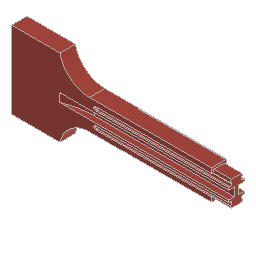
sentry (Autodesk Fusion 360 design; units mm, degrees)
Autodesk Fusion 360 part; units mm, degrees
sketch "base" plane through (0, 0, 0) normal (1, 0, 0) x (0, 1, 0)
  line L0 (0, 0) -> (0, 2.2125)
  line L1 (0, 0) -> (3.2, 0)
  line L2 (0, 2.2125) -> (1.175, 2.2125)
  line L3 (1.175, 2.2125) -> (1.175, 3.9625)
  line L4 (1.175, 3.9625) -> (0, 3.9625)
  line L5 (0, 3.9625) -> (0, 6.175)
  line L6 (0, 6.175) -> (3.2, 6.175)
  line L7 (3.2, 6.175) -> (3.2, 3.9625)
  line L8 (3.2, 3.9625) -> (2.025, 3.9625)
  line L9 (2.025, 3.9625) -> (2.025, 2.2125)
  line L10 (2.025, 2.2125) -> (3.2, 2.2125)
  line L11 (3.2, 2.2125) -> (3.2, 0)
  dimension "d1" = 2.2125
  dimension "d2" = 3.2
  dimension "d3" = 1.175
  dimension "d4" = 1.75
  dimension "d5" = 1.175
  dimension "d6" = 2.2125
  dimension "d7" = 3.2
  dimension "d8" = 2.2125
  dimension "d9" = 1.175
  dimension "d10" = 1.75
  dimension "d11" = 1.175
  constraint coincident L0.start L1.start
  constraint vertical L0
  constraint perpendicular L0 L1
  constraint perpendicular L0 L2
  constraint perpendicular L2 L3
  constraint perpendicular L3 L4
  constraint perpendicular L4 L5
  constraint perpendicular L5 L6
  constraint perpendicular L6 L7
  constraint perpendicular L7 L8
  constraint perpendicular L8 L9
  constraint perpendicular L9 L10
  measures "d1" distance of L0.start L0.end
  measures "d2" distance of L0.start L1.end
  measures "d3" distance of L0.end L2.end
  measures "d4" distance of L2.end L3.end
  measures "d5" distance of L3.end L4.end
  measures "d6" distance of L4.end L5.end
  measures "d7" distance of L5.end L6.end
  measures "d8" distance of L6.end L7.end
  measures "d9" distance of L7.end L8.end
  measures "d10" distance of L8.end L9.end
  measures "d11" distance of L9.end L10.end
extrude "Extrude1" add sketch "base" against normal blind 35
sketch "warding" plane through (0, 0, 0) normal (1, 0, 0) x (0, 1, 0)
  line L0 (0, 0) -> (3.2, 0) construction
  line L1 (0, 0) -> (0, 6.175) construction
  line L2 (0, 6.175) -> (3.2, 6.175) construction
  line L3 (0, 0) -> (0, 1) construction
  line L4 (3.2, 0) -> (3.2, 1) construction
  line L5 (0, 6.175) -> (0, 5.175) construction
  line L6 (3.2, 6.175) -> (3.2, 5.175) construction
  line L7 (0, 1) -> (0.6, 1)
  line L8 (3.2, 1) -> (2.6, 1)
  line L9 (0, 5.175) -> (0.6, 5.175)
  line L10 (3.2, 5.175) -> (2.6, 5.175)
  line L11 (0.6, 1) -> (0.6, 1.75)
  line L12 (2.6, 1) -> (2.6, 1.75)
  line L13 (0.6, 5.175) -> (0.6, 4.425)
  line L14 (2.6, 5.175) -> (2.6, 4.425)
  line L15 (0, 1) -> (0, 1.75)
  line L16 (3.2, 1) -> (3.2, 1.75)
  line L17 (0, 5.175) -> (0, 4.425)
  line L18 (3.2, 5.175) -> (3.2, 4.425)
  line L19 (0.6, 1.75) -> (0, 1.75)
  line L20 (3.2, 1.75) -> (2.6, 1.75)
  line L21 (0.6, 4.425) -> (0, 4.425)
  line L22 (2.6, 4.425) -> (3.2, 4.425)
  dimension "d14" = 3.2
  dimension "d15" = 6.175
  dimension "d16" = 3.2
  dimension "d17" = 1
  dimension "d18" = 1
  dimension "d19" = 1
  dimension "d20" = 1
  dimension "d21" = 0.6
  dimension "d22" = 0.6
  dimension "d23" = 0.6
  dimension "d24" = 0.6
  dimension "d25" = 0.75
  dimension "d26" = 0.75
  dimension "d27" = 0.75
  dimension "d28" = 0.75
  dimension "d29" = 0.75
  dimension "d30" = 0.75
  dimension "d31" = 0.75
  dimension "d32" = 0.75
  constraint coincident L0.start L1.start
  constraint horizontal L0
  constraint perpendicular L0 L1
  constraint perpendicular L1 L2
  constraint perpendicular L0 L3
  constraint perpendicular L0 L4
  constraint perpendicular L2 L5
  constraint perpendicular L2 L6
  constraint perpendicular L3 L7
  constraint perpendicular L4 L8
  constraint perpendicular L5 L9
  constraint perpendicular L6 L10
  constraint perpendicular L7 L11
  constraint perpendicular L8 L12
  constraint perpendicular L9 L13
  constraint perpendicular L10 L14
  constraint perpendicular L7 L15
  constraint perpendicular L8 L16
  constraint perpendicular L9 L17
  constraint perpendicular L10 L18
  measures "d14" distance of L0.start L0.end
  measures "d15" distance of L0.start L1.end
  measures "d16" distance of L1.end L2.end
  measures "d17" distance of L0.start L3.end
  measures "d18" distance of L0.end L4.end
  measures "d19" distance of L1.end L5.end
  measures "d20" distance of L2.end L6.end
  measures "d21" distance of L3.end L7.end
  measures "d22" distance of L4.end L8.end
  measures "d23" distance of L5.end L9.end
  measures "d24" distance of L6.end L10.end
  measures "d25" distance of L7.end L11.end
  measures "d26" distance of L8.end L12.end
  measures "d27" distance of L9.end L13.end
  measures "d28" distance of L10.end L14.end
  measures "d29" distance of L3.end L15.end
  measures "d30" distance of L4.end L16.end
  measures "d31" distance of L5.end L17.end
  measures "d32" distance of L6.end L18.end
extrude "Extrude2" cut sketch "warding" against normal blind 28
fillet "Fillet1" radius 0.325 8 edges at (-14, 0.6, 5.175) (-14, 0.6, 1.75) (-14, 0.6, 4.425) (-14, 0.6, 1) (-14, 2.6, 4.425) (-14, 2.6, 1) (-14, 2.6, 5.175) (-14, 2.6, 1.75)
fillet "Fillet2" radius 0.35 20 edges at (-28, 0.1375, 4.425) (-28, 0.5048, 4.5202) (-28, 0.6, 4.8) (-28, 0.5048, 5.0798) (-28, 0.1375, 5.175) (-28, 0.1375, 1) (-28, 0.5048, 1.0952) (-28, 0.6, 1.375) (-28, 0.5048, 1.6548) (-28, 0.1375, 1.75) (-28, 3.0625, 4.425) (-28, 2.6952, 4.5202) (-28, 2.6, 4.8) (-28, 2.6952, 5.0798) (-28, 3.0625, 5.175) (-28, 3.0625, 1) (-28, 2.6952, 1.0952) (-28, 2.6, 1.375) (-28, 2.6952, 1.6548) (-28, 3.0625, 1.75)
sketch "bow" plane through (-35, 0, 0) normal (-1, 0, 0) x (0, -1, 0)
  line L0 (-3.2, 0) -> (0, 0)
  line L1 (0, 0) -> (0, 2.2125)
  line L2 (0, 2.2125) -> (-1.175, 2.2125)
  line L3 (-1.175, 2.2125) -> (-1.175, 3.9625)
  line L4 (-1.175, 3.9625) -> (0, 3.9625)
  line L5 (0, 3.9625) -> (0, 6.175)
  line L6 (0, 6.175) -> (-3.2, 6.175)
  line L7 (-3.2, 6.175) -> (-3.2, 3.9625)
  line L8 (-3.2, 3.9625) -> (-2.025, 3.9625)
  line L9 (-2.025, 3.9625) -> (-2.025, 2.2125)
  line L10 (-2.025, 2.2125) -> (-3.2, 2.2125)
  line L11 (-3.2, 2.2125) -> (-3.2, 0)
  line L12 (0, 0) -> (0, 6.175) construction
  line L13 (0, 3.0875) -> (0, 11.0875)
  line L14 (0, 11.0875) -> (-3.2, 11.0875)
  line L15 (-3.2, 11.0875) -> (-3.2, -4.9125)
  line L16 (-3.2, -4.9125) -> (0, -4.9125)
  line L17 (0, -4.9125) -> (0, 6.175)
  dimension "d160" = 8
  dimension "d161" = 3.2
  dimension "d162" = 16
  dimension "d163" = 3.2
  constraint coincident L0.end L1.start
  constraint coincident L5.end L6.start
  constraint midpoint L12 L13.start
  constraint perpendicular L6 L13
  constraint perpendicular L13 L14
  constraint perpendicular L14 L15
  constraint perpendicular L15 L16
  measures "d160" distance of L13.start L13.end
  measures "d161" distance of L13.end L14.end
  measures "d162" distance of L14.end L15.end
  measures "d163" distance of L15.end L16.end
extrude "Extrude14" add sketch "bow" along normal blind 10
fillet "Fillet3" radius 6.25 2 edges at (-35, 1.6, 0) (-35, 1.6, 6.175)
fillet "Fillet4" radius 16.25 2 edges at (-35, 1.175, 3.0875) (-35, 2.025, 3.0875)
sketch "aws disc" plane through (0, 0, 0) normal (1, 0, 0) x (0, 1, 0)
  line L0 (0, 0) -> (1.6, 0) construction
  line L1 (1.6, 0) -> (1.6, 3.0875) construction
  line L2 (1.6, 3.0875) -> (1.6, 6.175) construction
  line L3 (1.6, 6.175) -> (0, 6.175) construction
  line L4 (1.6, 3.0875) -> (0, 3.0875) construction
  line L5 (1.6, 3.0875) -> (-0.2806, 3.9644) construction
  line L6 (1.6, 3.0875) -> (0, 3.0875) construction
  line L7 (-0.2806, 3.9644) -> (0.7502, 6.175)
  line L8 (1.6, 3.0875) -> (-0.2806, 2.2106) construction
  line L9 (1.6, 3.0875) -> (0, 3.0875) construction
  line L10 (-0.2806, 2.2106) -> (0.7502, 0)
  line L11 (1.6, 3.0875) -> (3.4806, 2.2106) construction
  line L12 (1.6, 3.0875) -> (3.4806, 3.9644) construction
  line L13 (3.4806, 3.9644) -> (2.4498, 6.175)
  line L14 (3.4806, 2.2106) -> (2.4498, 0)
  line L15 (0.7502, 6.175) -> (2.4498, 6.175)
  line L16 (0.7502, 0) -> (2.4498, 0)
  line L17 (-0.2806, 3.9644) -> (-0.2806, 2.2106)
  line L18 (3.4806, 3.9644) -> (3.4806, 2.2106)
  circle A0 centre (1.6, 3.0875) radius 4.25
  dimension "d37" = 1.6
  dimension "d38" = 3.0875
  dimension "d39" = 3.0875
  dimension "d40" = 1.6
  dimension "d41" = 1.6
  dimension "d42" = 25
  dimension "d43" = 2.075
  dimension "d44" = 25
  dimension "d45" = 2.075
  dimension "d46" = 8.5
  constraint coincident L0.start origin
  constraint horizontal L0
  constraint perpendicular L0 L1
  constraint parallel L1 L2
  constraint perpendicular L2 L3
  constraint perpendicular L1 L4
  constraint horizontal L6
  constraint coincident L3 L7.end
  constraint perpendicular L5 L7
  constraint horizontal L9
  constraint perpendicular L8 L10
  constraint equal L7 L10
  constraint parallel L5 L11
  constraint equal L5 L11
  constraint parallel L8 L12
  constraint equal L5 L12
  constraint perpendicular L12 L13
  constraint equal L7 L13
  constraint perpendicular L11 L14
  constraint equal L7 L14
  constraint coincident L1.end L2.start
  measures "d37" distance of L0.start L0.end
  measures "d38" distance of L0.end L1.end
  measures "d39" distance of L1.end L2.end
  measures "d40" distance of L2.end L3.end
  measures "d41" distance of L1.end L4.end
  measures "d42" angle of L5 L6
  measures "d43" distance of L1.end L5.end
  measures "d44" angle of L8 L9
  measures "d45" distance of L1.end L8.end
  measures "d46" diameter of A0
sketch "tip warding" plane through (0, 0, 0) normal (1, 0, 0) x (0, 1, 0)
  line L0 (0, 0) -> (3.2, 0)
  line L1 (1.6, 0) -> (1.6, 6.175) construction
  line L2 (1.6, 6.175) -> (0, 6.175)
  line L3 (1.6, 6.175) -> (3.2, 6.175)
  line L4 (0, 0) -> (0, 0.5)
  line L5 (3.2, 6.175) -> (3.2, 5.675)
  line L6 (0, 0.5) -> (3.2, 0.5)
  line L7 (3.2, 0.5) -> (3.2, 0)
  line L8 (3.2, 5.675) -> (0, 5.675)
  line L9 (0, 5.675) -> (0, 6.175)
  dimension "d47" = 3.2
  dimension "d48" = 6.175
  dimension "d49" = 1.6
  dimension "d50" = 1.6
  dimension "d51" = 0.5
  dimension "d52" = 0.5
  constraint coincident L0.start L4.start
  constraint horizontal L0
  constraint midpoint L0 L1.start
  constraint perpendicular L0 L1
  constraint perpendicular L1 L2
  constraint perpendicular L1 L3
  constraint perpendicular L0 L4
  constraint perpendicular L3 L5
  constraint perpendicular L4 L6
  constraint perpendicular L0 L7
  constraint perpendicular L5 L8
  constraint perpendicular L2 L9
  measures "d47" distance of L0.start L0.end
  measures "d48" distance of L1.start L1.end
  measures "d49" distance of L1.end L2.end
  measures "d50" distance of L1.end L3.end
  measures "d51" distance of L0.start L4.end
  measures "d52" distance of L3.end L5.end
extrude "Extrude3" cut sketch "tip warding" against normal blind 3.62
extrude "Extrude4" cut sketch "aws disc" against normal blind 3.62
sketch "Sketch12" plane through (0, 0, 0) normal (1, 0, 0) x (0, 1, 0)
  line L0 (0, 0) -> (1.6, 0) construction
  line L1 (1.6, 0) -> (1.6, 3.0875) construction
  line L2 (1.6, 3.0875) -> (0.6, 3.0875) construction
  line L3 (-0.6404, 3.4825) -> (3.8404, 2.6925) construction
  line L4 (-0.6404, 3.4825) -> (-0.0327, 6.9294)
  line L5 (3.8404, 2.6925) -> (3.2327, -0.7544)
  arc A0 (-0.6404, 3.4825) -> (-0.675, 3.0875) centre (1.6, 3.0875) ccw
  arc A1 (3.8404, 2.6925) -> (3.875, 3.0875) centre (1.6, 3.0875) ccw
  line L6 (3.875, 3.0875) -> (7.3391, 5.0875)
  line L7 (3.875, 3.0875) -> (1.6, 3.0875) construction
  line L8 (-0.675, 3.0875) -> (-4.1391, 1.0875)
  line L9 (-0.0327, 6.9294) -> (7.3391, 5.0875)
  line L10 (-4.1391, 1.0875) -> (3.2327, -0.7544)
  circle A2 centre (1.6, 3.0875) radius 7
  dimension "d197" = 1.6
  dimension "d198" = 3.0875
  dimension "d199" = 1
  dimension "d200" = 4.55
  dimension "d201" = 10
  dimension "d202" = 3.5
  dimension "d203" = 30
  dimension "d204" = 4
  dimension "d205" = 14
  constraint coincident L0.start origin
  constraint horizontal L0
  constraint perpendicular L0 L1
  constraint perpendicular L1 L2
  constraint midpoint L1.end L3
  constraint perpendicular L3 L4
  constraint perpendicular L3 L5
  constraint equal L4 L5
  constraint coincident L1.end L2.start
  constraint horizontal L1.end A0.end
  constraint collinear A0.end L1.end A1.end
  constraint horizontal L7
  constraint parallel L6 L8
  constraint equal L6 L8
  constraint concentric A1 A2
  measures "d197" distance of L0.start L0.end
  measures "d198" distance of L0.end L1.end
  measures "d199" distance of L1.end L2.end
  measures "d200" distance of L3.start L3.end
  measures "d201" angle of L2 L3
  measures "d202" distance of L3.start L4.end
  measures "d203" angle of L6 L7
  measures "d204" distance of A1.end L6.end
  measures "d205" diameter of A2
sketch "Sketch13" plane through (0, 0, 0) normal (1, 0, 0) x (0, 1, 0)
  circle A0 centre (1.6, 3.0875) radius 7
  line L0 (1.6, 3.0875) -> (0.6, 3.0875) construction
  line L1 (-0.6404, 3.4825) -> (3.8404, 2.6925) construction
  line L2 (-0.6404, 3.4825) -> (-0.0327, 6.9294)
  arc A1 (-0.6404, 3.4825) -> (-0.675, 3.0875) centre (1.6, 3.0875) ccw
  line L3 (-0.675, 3.0875) -> (-4.1391, 1.0875)
  line L4 (-0.675, 3.0875) -> (1.6, 3.0875) construction
  line L5 (3.8404, 2.6925) -> (3.2327, -0.7544)
  arc A2 (3.8404, 2.6925) -> (3.875, 3.0875) centre (1.6, 3.0875) ccw
  line L6 (3.875, 3.0875) -> (7.3391, 5.0875)
  line L7 (-0.0327, 6.9294) -> (7.3391, 5.0875)
  line L8 (-4.1391, 1.0875) -> (3.2327, -0.7544)
  dimension "d206" = 4.55
  dimension "d207" = 10
  dimension "d208" = 3.5
  dimension "d209" = 30
  dimension "d210" = 4
  constraint midpoint A0.centre L1
  constraint perpendicular L1 L2
  constraint coincident A0.centre L0.start
  constraint horizontal A0.centre A1.end
  constraint horizontal L4
  constraint perpendicular L1 L5
  constraint parallel L3 L6
  constraint equal L3 L6
  constraint collinear A0.centre A1.end A2.end
  constraint equal L2 L5
  measures "d206" distance of L1.start L1.end
  measures "d207" angle of L0 L1
  measures "d208" distance of L1.start L2.end
  measures "d209" angle of L3 L4
  measures "d210" distance of A1.end L3.end
sketch "Sketch14" plane through (0, 0, 0) normal (1, 0, 0) x (0, 1, 0)
  line L0 (1.6, 3.0875) -> (0.6, 3.0875) construction
  circle A0 centre (1.6, 3.0875) radius 7
  line L1 (-0.6404, 3.4825) -> (3.8404, 2.6925) construction
  line L2 (-0.6404, 3.4825) -> (-0.0327, 6.9294)
  arc A1 (-0.6404, 3.4825) -> (-0.675, 3.0875) centre (1.6, 3.0875) ccw
  line L3 (-0.675, 3.0875) -> (-4.1391, 1.0875)
  line L4 (-0.675, 3.0875) -> (1.6, 3.0875) construction
  line L5 (3.8404, 2.6925) -> (3.2327, -0.7544)
  arc A2 (3.8404, 2.6925) -> (3.875, 3.0875) centre (1.6, 3.0875) ccw
  line L6 (3.875, 3.0875) -> (7.3391, 5.0875)
  line L7 (-0.0327, 6.9294) -> (7.3391, 5.0875)
  line L8 (-4.1391, 1.0875) -> (3.2327, -0.7544)
  dimension "d211" = 4.55
  dimension "d212" = 10
  dimension "d213" = 3.5
  dimension "d214" = 30
  dimension "d215" = 4
  constraint midpoint L0.start L1
  constraint perpendicular L1 L2
  constraint coincident L0.start A0.centre
  constraint horizontal L0.start A1.end
  constraint horizontal L4
  constraint perpendicular L1 L5
  constraint equal L2 L5
  constraint collinear L0.start A1.end A2.end
  constraint parallel L3 L6
  constraint equal L3 L6
  measures "d211" distance of L1.start L1.end
  measures "d212" angle of L0 L1
  measures "d213" distance of L1.start L2.end
  measures "d214" angle of L3 L4
  measures "d215" distance of A1.end L3.end
sketch "Sketch15" plane through (0, 0, 0) normal (1, 0, 0) x (0, 1, 0)
  line L0 (1.6, 3.0875) -> (0.6, 3.0875) construction
  circle A0 centre (1.6, 3.0875) radius 7
  line L1 (-0.6404, 3.4825) -> (3.8404, 2.6925) construction
  line L2 (-0.6404, 3.4825) -> (-0.0327, 6.9294)
  arc A1 (-0.6404, 3.4825) -> (-0.675, 3.0875) centre (1.6, 3.0875) ccw
  line L3 (-0.675, 3.0875) -> (-4.1391, 1.0875)
  line L4 (-0.675, 3.0875) -> (1.6, 3.0875) construction
  line L5 (3.8404, 2.6925) -> (3.2327, -0.7544)
  arc A2 (3.8404, 2.6925) -> (3.875, 3.0875) centre (1.6, 3.0875) ccw
  line L6 (3.875, 3.0875) -> (7.3391, 5.0875)
  line L7 (-0.0327, 6.9294) -> (7.3391, 5.0875)
  line L8 (-4.1391, 1.0875) -> (3.2327, -0.7544)
  dimension "d216" = 4.55
  dimension "d217" = 10
  dimension "d218" = 3.5
  dimension "d219" = 30
  dimension "d220" = 4
  constraint midpoint L0.start L1
  constraint perpendicular L1 L2
  constraint coincident L0.start A0.centre
  constraint horizontal L0.start A1.end
  constraint horizontal L4
  constraint perpendicular L1 L5
  constraint equal L2 L5
  constraint collinear A1.end L0.start A2.end
  constraint parallel L3 L6
  constraint equal L3 L6
  measures "d216" distance of L1.start L1.end
  measures "d217" angle of L0 L1
  measures "d218" distance of L1.start L2.end
  measures "d219" angle of L3 L4
  measures "d220" distance of A1.end L3.end
sketch "Sketch16" plane through (0, 0, 0) normal (1, 0, 0) x (0, 1, 0)
  line L0 (1.6, 3.0875) -> (0.6, 3.0875) construction
  circle A0 centre (1.6, 3.0875) radius 7
  line L1 (-0.6404, 3.4825) -> (3.8404, 2.6925) construction
  line L2 (-0.6404, 3.4825) -> (-0.0327, 6.9294)
  line L3 (3.8404, 2.6925) -> (3.2327, -0.7544)
  arc A1 (-0.6404, 3.4825) -> (-0.675, 3.0875) centre (1.6, 3.0875) ccw
  arc A2 (3.8404, 2.6925) -> (3.875, 3.0875) centre (1.6, 3.0875) ccw
  line L4 (-0.675, 3.0875) -> (-4.1391, 1.0875)
  line L5 (-0.675, 3.0875) -> (1.6, 3.0875) construction
  line L6 (3.875, 3.0875) -> (7.3391, 5.0875)
  line L7 (7.3391, 5.0875) -> (-0.0327, 6.9294)
  line L8 (-4.1391, 1.0875) -> (3.2327, -0.7544)
  dimension "d221" = 4.55
  dimension "d222" = 3.5
  dimension "d223" = 30
  dimension "d224" = 4
  dimension "d225" = 10
  constraint perpendicular L1 L2
  constraint perpendicular L1 L3
  constraint equal L2 L3
  constraint midpoint L1 L0.start
  constraint coincident L0.start A0.centre
  constraint collinear L0.start A1.end A2.end
  constraint horizontal L5
  constraint parallel L4 L6
  constraint equal L4 L6
  constraint midpoint L0.start L1
  measures "d221" distance of L1.start L1.end
  measures "d222" distance of L1.start L2.end
  measures "d223" angle of L4 L5
  measures "d224" distance of A1.end L4.end
  measures "d225" angle of L1 L5
sketch "Sketch17" plane through (0, 0, 0) normal (1, 0, 0) x (0, 1, 0)
  line L0 (1.6, 3.0875) -> (0.6, 3.0875) construction
  circle A0 centre (1.6, 3.0875) radius 7
  line L1 (-0.6404, 3.4825) -> (3.8404, 2.6925) construction
  line L2 (-0.6404, 3.4825) -> (-0.0327, 6.9294)
  line L3 (3.8404, 2.6925) -> (3.2327, -0.7544)
  arc A1 (-0.6404, 3.4825) -> (-0.675, 3.0875) centre (1.6, 3.0875) ccw
  arc A2 (3.8404, 2.6925) -> (3.875, 3.0875) centre (1.6, 3.0875) ccw
  line L4 (-0.675, 3.0875) -> (-4.1391, 1.0875)
  line L5 (-0.675, 3.0875) -> (1.6, 3.0875) construction
  line L6 (3.875, 3.0875) -> (7.3391, 5.0875)
  line L7 (-0.0327, 6.9294) -> (7.3391, 5.0875)
  line L8 (3.2327, -0.7544) -> (-4.1391, 1.0875)
  dimension "d226" = 4.55
  dimension "d227" = 3.5
  dimension "d228" = 30
  dimension "d229" = 4
  dimension "d230" = 10
  constraint perpendicular L1 L2
  constraint perpendicular L1 L3
  constraint equal L2 L3
  constraint midpoint L1 L0.start
  constraint horizontal L0.start A1.end
  constraint coincident L0.start A0.centre
  constraint collinear A1.end L0.start A2.end
  constraint horizontal L5
  constraint parallel L4 L6
  constraint equal L4 L6
  constraint midpoint L0.start L1
  measures "d226" distance of L1.start L1.end
  measures "d227" distance of L1.start L2.end
  measures "d228" angle of L4 L5
  measures "d229" distance of A1.end L4.end
  measures "d230" angle of L1 L5
sketch "Sketch18" plane through (0, 0, 0) normal (1, 0, 0) x (0, 1, 0)
  line L0 (1.6, 3.0875) -> (0.6, 3.0875) construction
  circle A0 centre (1.6, 3.0875) radius 7
  line L1 (-0.6404, 3.4825) -> (3.8404, 2.6925) construction
  line L2 (-0.6404, 3.4825) -> (-0.0327, 6.9294)
  line L3 (3.8404, 2.6925) -> (3.2327, -0.7544)
  arc A1 (-0.6404, 3.4825) -> (-0.675, 3.0875) centre (1.6, 3.0875) ccw
  arc A2 (3.8404, 2.6925) -> (3.875, 3.0875) centre (1.6, 3.0875) ccw
  line L4 (-0.675, 3.0875) -> (-4.1391, 1.0875)
  line L5 (-0.675, 3.0875) -> (1.6, 3.0875) construction
  line L6 (3.875, 3.0875) -> (7.3391, 5.0875)
  line L7 (7.3391, 5.0875) -> (-0.0327, 6.9294)
  line L8 (-4.1391, 1.0875) -> (3.2327, -0.7544)
  dimension "d231" = 4.55
  dimension "d232" = 3.5
  dimension "d233" = 30
  dimension "d234" = 4
  dimension "d235" = 10
  constraint perpendicular L1 L2
  constraint perpendicular L1 L3
  constraint equal L2 L3
  constraint midpoint L1 L0.start
  constraint horizontal L0.start A1.end
  constraint coincident L0.start A0.centre
  constraint collinear L0.start A1.end A2.end
  constraint horizontal L5
  constraint parallel L4 L6
  constraint equal L4 L6
  constraint midpoint L0.start L1
  measures "d231" distance of L1.start L1.end
  measures "d232" distance of L1.start L2.end
  measures "d233" angle of L4 L5
  measures "d234" distance of A1.end L4.end
  measures "d235" angle of L1 L5
sketch "Sketch19" plane through (0, 0, 0) normal (1, 0, 0) x (0, 1, 0)
  line L0 (1.6, 3.0875) -> (0.6, 3.0875) construction
  circle A0 centre (1.6, 3.0875) radius 7
  line L1 (-0.6404, 3.4825) -> (3.8404, 2.6925) construction
  line L2 (-0.6404, 3.4825) -> (-0.0327, 6.9294)
  line L3 (3.8404, 2.6925) -> (3.2327, -0.7544)
  arc A1 (-0.6404, 3.4825) -> (-0.675, 3.0875) centre (1.6, 3.0875) ccw
  arc A2 (3.8404, 2.6925) -> (3.875, 3.0875) centre (1.6, 3.0875) ccw
  line L4 (-0.675, 3.0875) -> (-4.1391, 1.0875)
  line L5 (-0.675, 3.0875) -> (1.6, 3.0875) construction
  line L6 (3.875, 3.0875) -> (7.3391, 5.0875)
  line L7 (7.3391, 5.0875) -> (-0.0327, 6.9294)
  line L8 (-4.1391, 1.0875) -> (3.2327, -0.7544)
  dimension "d236" = 4.55
  dimension "d237" = 3.5
  dimension "d238" = 30
  dimension "d239" = 4
  dimension "d240" = 10
  constraint perpendicular L1 L2
  constraint perpendicular L1 L3
  constraint equal L2 L3
  constraint midpoint L1 L0.start
  constraint horizontal L0.start A1.end
  constraint coincident L0.start A0.centre
  constraint collinear L0.start A1.end A2.end
  constraint horizontal L5
  constraint parallel L4 L6
  constraint equal L4 L6
  constraint midpoint L0.start L1
  measures "d236" distance of L1.start L1.end
  measures "d237" distance of L1.start L2.end
  measures "d238" angle of L4 L5
  measures "d239" distance of A1.end L4.end
  measures "d240" angle of L1 L5
sketch "Sketch20" plane through (0, 0, 0) normal (1, 0, 0) x (0, 1, 0)
  line L0 (1.6, 3.0875) -> (0.6, 3.0875) construction
  circle A0 centre (1.6, 3.0875) radius 7
  line L1 (-0.6404, 3.4825) -> (3.8404, 2.6925) construction
  line L2 (-0.6404, 3.4825) -> (-0.0327, 6.9294)
  line L3 (3.8404, 2.6925) -> (3.2327, -0.7544)
  arc A1 (-0.6404, 3.4825) -> (-0.675, 3.0875) centre (1.6, 3.0875) ccw
  arc A2 (3.8404, 2.6925) -> (3.875, 3.0875) centre (1.6, 3.0875) ccw
  line L4 (-0.675, 3.0875) -> (-4.1391, 1.0875)
  line L5 (-0.675, 3.0875) -> (1.6, 3.0875) construction
  line L6 (3.875, 3.0875) -> (7.3391, 5.0875)
  line L7 (-4.1391, 1.0875) -> (3.2327, -0.7544)
  line L8 (7.3391, 5.0875) -> (-0.0327, 6.9294)
  dimension "d241" = 4.55
  dimension "d242" = 3.5
  dimension "d243" = 30
  dimension "d244" = 4
  dimension "d245" = 10
  constraint perpendicular L1 L2
  constraint perpendicular L1 L3
  constraint equal L2 L3
  constraint midpoint L1 L0.start
  constraint horizontal L0.start A1.end
  constraint coincident L0.start A0.centre
  constraint collinear A1.end L0.start A2.end
  constraint horizontal L5
  constraint parallel L4 L6
  constraint equal L4 L6
  constraint midpoint L0.start L1
  measures "d241" distance of L1.start L1.end
  measures "d242" distance of L1.start L2.end
  measures "d243" angle of L4 L5
  measures "d244" distance of A1.end L4.end
  measures "d245" angle of L1 L5
extrude "1" cut sketch "Sketch12" along normal mid plane 2.6 from surface at -4.92
extrude "2" cut sketch "Sketch13" along normal mid plane 2.6 from surface at -6.87
extrude "3" cut sketch "Sketch14" along normal mid plane 2.6 from surface at -8.82
extrude "4" cut sketch "Sketch15" along normal mid plane 2.6 from surface at -10.77
extrude "5" cut sketch "Sketch16" along normal mid plane 2.6 from surface at -12.72
extrude "6" cut sketch "Sketch17" along normal mid plane 2.6 from surface at -14.67
extrude "7" cut sketch "Sketch18" along normal mid plane 2.6 from surface at -16.62
extrude "8" cut sketch "Sketch19" along normal mid plane 2.6 from surface at -18.57
extrude "9" cut sketch "Sketch20" along normal mid plane 2.6 from surface at -20.52
equation "d5 = d3"
equation "d6 = d1"
equation "d7 = d2"
equation "d8 = d1"
equation "d9 = d3"
equation "d10 = d4"
equation "d11 = d3"
equation "d14 = d2"
equation "d15 = d1 * 2 + d4"
equation "d16 = d2"
equation "d18 = d17"
equation "d19 = d17"
equation "d20 = d17"
equation "d22 = d21"
equation "d23 = d21"
equation "d24 = d21"
equation "d26 = d25"
equation "d27 = d25"
equation "d28 = d25"
equation "d29 = d25"
equation "d30 = d25"
equation "d31 = d25"
equation "d32 = d25"
equation "d37 = d2 / 2"
equation "d38 = d1 + d4 / 2"
equation "d39 = d38"
equation "d40 = d37"
equation "d41 = d37"
equation "d43 = ( 4.15 / 2 ) * 1 mm"
equation "d44 = d42"
equation "d45 = d43"
equation "d47 = d2"
equation "d48 = d1 * 2 + d4"
equation "d49 = d2 / 2"
equation "d50 = d49"
equation "d52 = d51"
equation "d53 = -3.62 mm"
equation "d55 = d53"
equation "offset = 3.62 mm - 0.65 mm"
equation "spacing = 1.95 mm"
equation "width = 1.3 mm"
equation "d129 = -offset - ( spacing * 1 )"
equation "d130 = width"
equation "d132 = -offset - ( spacing * 2 )"
equation "d133 = width"
equation "d135 = -offset - ( spacing * 3 )"
equation "d136 = width"
equation "d138 = -offset - ( spacing * 4 )"
equation "d139 = width"
equation "d141 = -offset - ( spacing * 5 )"
equation "d142 = width"
equation "d144 = -offset - ( spacing * 6 )"
equation "d145 = width"
equation "d147 = -offset - ( spacing * 7 )"
equation "d148 = width"
equation "d150 = -offset - ( spacing * 8 )"
equation "d151 = width"
equation "d153 = -offset - ( spacing * 9 )"
equation "d154 = width"
equation "d161 = d2"
equation "d162 = d160 * 2"
equation "d163 = d161"
equation "pos_1 = round($1)"
equation "cut_1 = if(pos_1 == 1; 10 deg; if(pos_1 == 2; 28 deg; if(pos_1 == 3; 46 deg; if(pos_1 == 4; 64 deg; if(pos_1 == 5; 82 deg; 100 deg)))))"
equation "pos_2 = round($2)"
equation "cut_2 = if(pos_2 == 1; 10 deg; if(pos_2 == 2; 28 deg; if(pos_2 == 3; 46 deg; if(pos_2 == 4; 64 deg; if(pos_2 == 5; 82 deg; 100 deg)))))"
equation "pos_3 = round($3)"
equation "cut_3 = if(pos_3 == 1; 10 deg; if(pos_3 == 2; 28 deg; if(pos_3 == 3; 46 deg; if(pos_3 == 4; 64 deg; if(pos_3 == 5; 82 deg; 100 deg)))))"
equation "pos_4 = round($4)"
equation "cut_4 = if(pos_4 == 1; 10 deg; if(pos_4 == 2; 28 deg; if(pos_4 == 3; 46 deg; if(pos_4 == 4; 64 deg; if(pos_4 == 5; 82 deg; 100 deg)))))"
equation "pos_5 = round($5)"
equation "cut_5 = if(pos_5 == 1; 10 deg; if(pos_5 == 2; 28 deg; if(pos_5 == 3; 46 deg; if(pos_5 == 4; 64 deg; if(pos_5 == 5; 82 deg; 100 deg)))))"
equation "pos_6 = round($6)"
equation "cut_6 = if(pos_6 == 1; 10 deg; if(pos_6 == 2; 28 deg; if(pos_6 == 3; 46 deg; if(pos_6 == 4; 64 deg; if(pos_6 == 5; 82 deg; 100 deg)))))"
equation "pos_7 = round($7)"
equation "cut_7 = if(pos_7 == 1; 10 deg; if(pos_7 == 2; 28 deg; if(pos_7 == 3; 46 deg; if(pos_7 == 4; 64 deg; if(pos_7 == 5; 82 deg; 100 deg)))))"
equation "pos_8 = round($8)"
equation "cut_8 = if(pos_8 == 1; 10 deg; if(pos_8 == 2; 28 deg; if(pos_8 == 3; 46 deg; if(pos_8 == 4; 64 deg; if(pos_8 == 5; 82 deg; 100 deg)))))"
equation "pos_9 = round($9)"
equation "cut_9 = if(pos_9 == 1; 10 deg; if(pos_9 == 2; 28 deg; if(pos_9 == 3; 46 deg; if(pos_9 == 4; 64 deg; if(pos_9 == 5; 82 deg; 100 deg)))))"
equation "d197 = d2 * 0.5"
equation "d198 = d1 + 0.5 * d4"
equation "d200 = 2.275 mm * 2"
equation "d201 = cut_1"
equation "d206 = d200"
equation "d207 = cut_2"
equation "d208 = d202"
equation "d209 = d203"
equation "d210 = d204"
equation "d211 = d200"
equation "d212 = cut_3"
equation "d213 = d202"
equation "d214 = d203"
equation "d215 = d204"
equation "d216 = d200"
equation "d217 = cut_4"
equation "d218 = d202"
equation "d219 = d203"
equation "d220 = d204"
equation "d221 = d200"
equation "d222 = d202"
equation "d223 = d203"
equation "d224 = d204"
equation "d225 = cut_5"
equation "d226 = d200"
equation "d227 = d202"
equation "d228 = d203"
equation "d229 = d204"
equation "d230 = cut_6"
equation "d231 = d200"
equation "d232 = d202"
equation "d233 = d203"
equation "d234 = d204"
equation "d235 = cut_7"
equation "d236 = d200"
equation "d237 = d202"
equation "d238 = d203"
equation "d239 = d204"
equation "d240 = cut_8"
equation "d241 = d200"
equation "d242 = d202"
equation "d243 = d203"
equation "d244 = d204"
equation "d245 = cut_9"
named bodies: "key"
